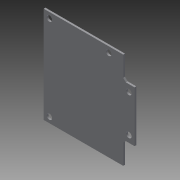
# Autodesk Inventor part: Pixy
Saved by Autodesk Inventor 2015 (Build 190159000, 159)
## iProperties
Created: 2016-02-22
Part Number: Pixy
Material: Generic
Document SubType Name: Modeling
Designer: James Yelland
Density: 1 g/cm^3
Appearance: Default
Author: James Yelland
Autodesk Inventor part; units mm, degrees
ref_plane "YZ Plane" through (0, 0, 0) normal (1, 0, 0) x (0, 1, 0)
ref_plane "XZ Plane" through (0, 0, 0) normal (0, 1, 0) x (-1, 0, 0)
ref_plane "XY Plane" through (0, 0, 0) normal (0, 0, 1) x (1, 0, 0)
sketch "Sketch1" plane through (0, 0, 0) normal (0, 1, 0) x (-1, 0, 0)
  line L0 (50.8, 26.924) -> (50.8, -26.924)
  line L1 (6.35, 26.924) -> (6.35, 15.724)
  line L2 (4.85, 14.224) -> (0, 14.224)
  line L3 (6.35, 26.924) -> (50.8, 26.924)
  line L4 (0, -14.224) -> (4.85, -14.224)
  line L5 (6.35, -15.724) -> (6.35, -26.924)
  line L6 (0, 0) -> (0, 14.224)
  line L7 (0, 0) -> (0, -14.224)
  line L8 (6.35, -26.924) -> (50.8, -26.924)
  line L9 (4.85, 14.224) -> (6.35, 15.724)
  line L10 (4.85, -14.224) -> (6.35, -15.724)
  line L11 (50.8, 26.924) -> (50.8, 23.749)
  circle A0 centre (47.625, 23.749) radius 1.524
  line L12 (50.8, -26.924) -> (50.8, -23.749)
  circle A1 centre (47.625, -23.749) radius 1.524
  line L13 (6.35, 26.924) -> (14.478, 26.924)
  circle A2 centre (14.478, 23.749) radius 1.524
  circle A3 centre (3.175, -10.414) radius 1.524
  circle A4 centre (3.175, 10.414) radius 1.524
  point P0 (6.35, 14.224)
  point P1 (6.35, -14.224)
  constraints: 28 end point, 7 point on line, 5 centre point, 3 vertical, 2 perpendicular, 1 horizontal
extrude "Extrusion1" add sketch "Sketch1" along normal blind 1
body "Solid1"
